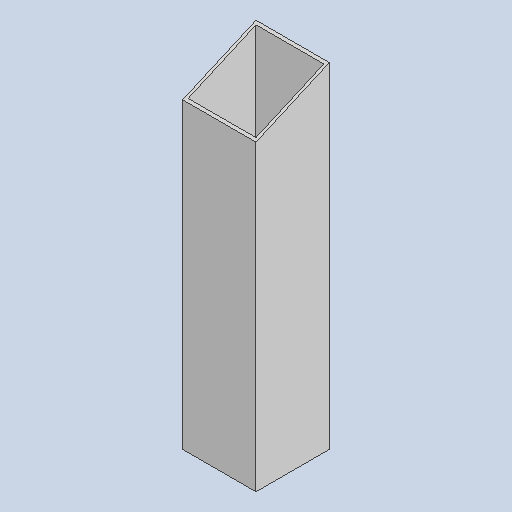
# Autodesk Inventor part: PRS 9681 leg tube_D1200
Saved by Autodesk Inventor 2026.2 (Build 302298000, 298)
## iProperties
Created: 2026-06-11
Part Number: PRS 9681 leg tube_D1200
Material: Generic
Document SubType Name: Modeling
Designer: admin
Density: 1 g/cm^3
Appearance: Default
Author: admin
Autodesk Inventor part; units mm, degrees
ref_plane "YZ Plane" through (0, 0, 0) normal (1, 0, 0) x (0, 1, 0)
ref_plane "XZ Plane" through (0, 0, 0) normal (0, 1, 0) x (-1, 0, 0)
ref_plane "XY Plane" through (0, 0, 0) normal (0, 0, 1) x (1, 0, 0)
sketch "Sketch1" plane through (0, 0, 0) normal (0, 1, 0) x (-1, 0, 0)
  line L0 (40, -40) -> (-40, -40)
  line L1 (-40, -40) -> (-40, 40)
  line L2 (-40, 40) -> (40, 40)
  line L3 (40, 40) -> (40, -40)
  line L4 (40, -40) -> (-40, 40) construction
  line L5 (-40, -40) -> (40, 40) construction
  line L6 (-37, -37) -> (37, -37)
  line L7 (37, -37) -> (37, 37)
  line L8 (37, 37) -> (-37, 37)
  line L9 (-37, 37) -> (-37, -37)
  point P0 (0, 0)
  dimension "d0" = 3
  dimension "d1" = 80
  constraints: 20 end point, 4 parallel, 3 perpendicular, 2 midpoint, 1 horizontal, 3 other
  measures "d0" distance between parallel lines of L0 L6
  measures "d1" distance of L0.start L0.end
extrude "Extrusion1" add sketch "Sketch1" along normal blind 365.45
sketch "Sketch2" plane through (0, 0, 0) normal (1, 0, 0) x (0, 1, 0)
  line L0 (0, 40) -> (0, -40) construction
  line L1 (0, -40) -> (365.45, -40) projected
  line L2 (365.45, 40) -> (365.45, -40) projected
  line L3 (0, 40) -> (365.45, 40) projected
  line L4 (0, -40) -> (365.45, -40) projected
  line L5 (365.45, -40) -> (330.2832, 40)
  point P0 (0, 0)
  dimension "d4" = 23.73
  constraints: 2 end point, 1 point on line
  measures "d4" angle of L5 L2
extrude "Extrusion2" cut sketch "Sketch2" along normal through all both and the other way through all
equation "\"d1\" = Legs_Tube_dim"
equation "\"d4\" = Legs_Tube_cut_angle"
equation "\"Legs_Tube_dim\" = 80"
body "Solid1"
